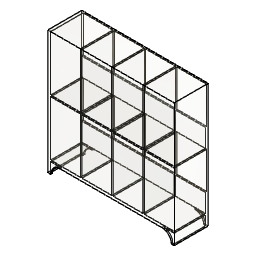
sorted_smarties_collector (Autodesk Fusion 360 design; units mm, degrees)
Autodesk Fusion 360 part; units mm, degrees
note: some values were not read from the file. Set by a fixed rule: which sketch regions a step uses.
sketch "Sorted Smarties Collector" plane through (0, 0, 0) normal (0, 1, 0) x (1, 0, 0)
  line L0 (0, 0) -> (268, 0)
  line L1 (268, 0) -> (268, -262)
  line L2 (268, -262) -> (0, -262)
  line L3 (0, -262) -> (0, 0)
  dimension "d1" = 268
  dimension "d41" = 262
  constraint horizontal L0
  constraint vertical L1
  constraint horizontal L2
  constraint vertical L3
  constraint coincident L0.start L3.end
  measures "d1" distance of L0.start L0.end
  measures "d41" distance of L0.end L1.end
extrude "Extrude1" add sketch "Sorted Smarties Collector" along normal blind 3
sketch "Smartie Collectors" plane through (0, 3, 0) normal (0, 1, 0) x (-1, 0, 0)
  line L0 (0, 262) -> (-268, 262)
  line L1 (-268, 262) -> (-268, 0)
  line L2 (-268, 0) -> (0, 0)
  line L3 (0, 0) -> (0, 262)
  line L4 (-265, 259) -> (-201.75, 259)
  line L5 (-201.75, 259) -> (-201.75, 142.5)
  line L6 (-201.75, 142.5) -> (-265, 142.5)
  line L7 (-265, 142.5) -> (-265, 259)
  line L8 (-198.75, 259) -> (-135.5, 259)
  line L9 (-135.5, 259) -> (-135.5, 142.5)
  line L10 (-135.5, 142.5) -> (-198.75, 142.5)
  line L11 (-198.75, 142.5) -> (-198.75, 259)
  line L12 (-132.5, 259) -> (-69.25, 259)
  line L13 (-69.25, 259) -> (-69.25, 142.5)
  line L14 (-69.25, 142.5) -> (-132.5, 142.5)
  line L15 (-132.5, 142.5) -> (-132.5, 259)
  line L16 (-66.25, 259) -> (-3, 259)
  line L17 (-3, 259) -> (-3, 142.5)
  line L18 (-3, 142.5) -> (-66.25, 142.5)
  line L19 (-66.25, 142.5) -> (-66.25, 259)
  line L20 (-265, 139.5) -> (-201.75, 139.5)
  line L21 (-201.75, 139.5) -> (-201.75, 23)
  line L22 (-201.75, 23) -> (-265, 23)
  line L23 (-265, 23) -> (-265, 139.5)
  line L24 (-198.75, 139.5) -> (-135.5, 139.5)
  line L25 (-135.5, 139.5) -> (-135.5, 23)
  line L26 (-135.5, 23) -> (-198.75, 23)
  line L27 (-198.75, 23) -> (-198.75, 139.5)
  line L28 (-132.5, 139.5) -> (-69.25, 139.5)
  line L29 (-69.25, 139.5) -> (-69.25, 23)
  line L30 (-69.25, 23) -> (-132.5, 23)
  line L31 (-132.5, 23) -> (-132.5, 139.5)
  line L32 (-66.25, 139.5) -> (-3, 139.5)
  line L33 (-3, 139.5) -> (-3, 23)
  line L34 (-3, 23) -> (-66.25, 23)
  line L35 (-66.25, 23) -> (-66.25, 139.5)
  line L36 (-265, 0) -> (-3, 0)
  line L37 (-3, 0) -> (-3, 20)
  line L38 (-3, 20) -> (-265, 20)
  line L39 (-265, 20) -> (-265, 0)
  dimension "d51" = 3
  dimension "d52" = 3
  dimension "d53" = 3
  dimension "d54" = 20
  dimension "d55" = 3
  dimension "d56" = 3
  dimension "d57" = 3
  dimension "d58" = 3
  dimension "d59" = 3
  dimension "d60" = 116.5
  dimension "d61" = 116.5
  dimension "d62" = 63.25
  dimension "d63" = 63.25
  dimension "d64" = 63.25
  dimension "d65" = 63.25
  constraint horizontal L4
  constraint vertical L5
  constraint horizontal L6
  constraint vertical L7
  constraint horizontal L8
  constraint vertical L9
  constraint horizontal L10
  constraint vertical L11
  constraint horizontal L12
  constraint vertical L13
  constraint horizontal L14
  constraint vertical L15
  constraint horizontal L16
  constraint vertical L17
  constraint horizontal L18
  constraint vertical L19
  constraint horizontal L20
  constraint vertical L21
  constraint horizontal L22
  constraint vertical L23
  constraint horizontal L24
  constraint vertical L25
  constraint horizontal L26
  constraint vertical L27
  constraint horizontal L28
  constraint vertical L29
  constraint horizontal L30
  constraint vertical L31
  constraint horizontal L32
  constraint vertical L33
  constraint horizontal L34
  constraint vertical L35
  constraint collinear L4 L8
  constraint collinear L8 L12
  constraint collinear L12 L16
  constraint collinear L6 L10
  constraint collinear L10 L14
  constraint collinear L14 L18
  constraint collinear L22 L26
  constraint collinear L26 L30
  constraint collinear L30 L34
  constraint collinear L20 L24
  constraint collinear L24 L28
  constraint collinear L28 L32
  constraint horizontal L36
  constraint vertical L37
  constraint horizontal L38
  constraint vertical L39
  constraint coincident L2 L36.start
  constraint collinear L23 L39
  constraint collinear L7 L23
  constraint collinear L5 L21
  constraint collinear L11 L27
  constraint collinear L9 L25
  constraint collinear L15 L31
  constraint collinear L13 L29
  constraint collinear L19 L35
  constraint collinear L17 L33
  constraint collinear L33 L37
  measures "d51" distance of L0 L4
  measures "d52" distance of L6 L20
  measures "d53" distance of L22 L38
  measures "d54" distance of L36 L38
  measures "d55" distance of L5 L11
  measures "d56" distance of L9 L15
  measures "d57" distance of L13 L19
  measures "d58" distance of L1 L7
  measures "d59" distance of L3 L17
  measures "d60" distance of L16.end L17.end
  measures "d61" distance of L32.end L33.end
  measures "d62" distance of L4.start L4.end
  measures "d63" distance of L8.start L8.end
  measures "d64" distance of L12.start L12.end
  measures "d65" distance of L16.start L16.end
extrude "Extrude2" add sketch "Smartie Collectors" along normal blind 69 contours L0 L1 L2 L3 L37 L38 L39
sketch "Front Panel" plane through (268, 0, 0) normal (1, 0, 0) x (0, 1, 0)
  line L0 (0, 262) -> (0, 0)
  line L1 (0, 0) -> (72, 0)
  line L2 (72, 0) -> (72, 262)
  line L3 (72, 262) -> (0, 262)
  line L4 (72, 262) -> (69, 262)
  line L5 (69, 262) -> (69, 0)
  line L6 (69, 0) -> (72, 0)
  line L7 (72, 0) -> (72, 262)
  dimension "d66" = 3
  constraint horizontal L4
  constraint vertical L5
  constraint horizontal L6
  constraint vertical L7
  constraint coincident L1 L5.end
  constraint coincident L2.end L3.start
  measures "d66" distance of L5.end L1.end
extrude "Extrude3" add sketch "Front Panel" against normal blind 268 contours L1 L2 L3 L4 L5 L6 L7
sketch "Front Openings" plane through (0, 72, 0) normal (0, 1, 0) x (-1, 0, 0)
  line L0 (-268, 0) -> (0, 0)
  line L1 (0, 0) -> (0, 262)
  line L2 (0, 262) -> (-268, 262)
  line L3 (-268, 262) -> (-268, 0)
  line L4 (0, 262) -> (-268, 262)
  line L5 (-198.75, 259) -> (-135.5, 259)
  line L6 (-265, 259) -> (-201.75, 259)
  line L7 (-201.75, 142.5) -> (-265, 142.5)
  line L8 (-265, 139.5) -> (-201.75, 139.5)
  line L9 (-201.75, 23) -> (-265, 23)
  line L10 (-135.5, 23) -> (-198.75, 23)
  line L11 (-69.25, 23) -> (-132.5, 23)
  line L12 (-3, 23) -> (-66.25, 23)
  line L13 (-132.5, 139.5) -> (-69.25, 139.5)
  line L14 (-198.75, 139.5) -> (-135.5, 139.5)
  line L15 (-135.5, 142.5) -> (-198.75, 142.5)
  line L16 (-69.25, 142.5) -> (-132.5, 142.5)
  line L17 (-3, 142.5) -> (-66.25, 142.5)
  line L18 (-66.25, 139.5) -> (-3, 139.5)
  line L19 (-132.5, 259) -> (-69.25, 259)
  line L20 (-66.25, 259) -> (-3, 259)
  line L21 (-3, 20) -> (-265, 20)
  line L22 (-3, 0) -> (-3, 20)
  line L23 (-265, 20) -> (-265, 0)
  line L24 (-265, 23) -> (-265, 139.5)
  line L25 (-201.75, 139.5) -> (-201.75, 23)
  line L26 (-198.75, 23) -> (-198.75, 139.5)
  line L27 (-135.5, 139.5) -> (-135.5, 23)
  line L28 (-132.5, 23) -> (-132.5, 139.5)
  line L29 (-69.25, 139.5) -> (-69.25, 23)
  line L30 (-66.25, 23) -> (-66.25, 139.5)
  line L31 (-3, 139.5) -> (-3, 23)
  line L32 (-265, 142.5) -> (-265, 259)
  line L33 (-201.75, 259) -> (-201.75, 142.5)
  line L34 (-198.75, 142.5) -> (-198.75, 259)
  line L35 (-135.5, 259) -> (-135.5, 142.5)
  line L36 (-132.5, 142.5) -> (-132.5, 259)
  line L37 (-69.25, 259) -> (-69.25, 142.5)
  line L38 (-66.25, 142.5) -> (-66.25, 259)
  line L39 (-3, 259) -> (-3, 142.5)
  line L40 (-265, 259) -> (-201.75, 259)
  line L41 (-201.75, 259) -> (-201.75, 181.3333)
  line L42 (-201.75, 181.3333) -> (-265, 181.3333)
  line L43 (-265, 181.3333) -> (-265, 259)
  line L44 (-198.75, 259) -> (-135.5, 259)
  line L45 (-135.5, 259) -> (-135.5, 181.3333)
  line L46 (-135.5, 181.3333) -> (-198.75, 181.3333)
  line L47 (-198.75, 181.3333) -> (-198.75, 259)
  line L48 (-132.5, 259) -> (-69.25, 259)
  line L49 (-69.25, 259) -> (-69.25, 181.3333)
  line L50 (-69.25, 181.3333) -> (-132.5, 181.3333)
  line L51 (-132.5, 181.3333) -> (-132.5, 259)
  line L52 (-66.25, 259) -> (-3, 259)
  line L53 (-3, 259) -> (-3, 181.3333)
  line L54 (-3, 181.3333) -> (-66.25, 181.3333)
  line L55 (-66.25, 181.3333) -> (-66.25, 259)
  line L56 (-265, 139.5) -> (-201.75, 139.5)
  line L57 (-201.75, 139.5) -> (-201.75, 61.8333)
  line L58 (-201.75, 61.8333) -> (-265, 61.8333)
  line L59 (-265, 61.8333) -> (-265, 139.5)
  line L60 (-198.75, 139.5) -> (-135.5, 139.5)
  line L61 (-135.5, 139.5) -> (-135.5, 61.8333)
  line L62 (-135.5, 61.8333) -> (-198.75, 61.8333)
  line L63 (-198.75, 61.8333) -> (-198.75, 139.5)
  line L64 (-132.5, 139.5) -> (-69.25, 139.5)
  line L65 (-69.25, 139.5) -> (-69.25, 61.8333)
  line L66 (-69.25, 61.8333) -> (-132.5, 61.8333)
  line L67 (-132.5, 61.8333) -> (-132.5, 139.5)
  line L68 (-66.25, 139.5) -> (-3, 139.5)
  line L69 (-3, 139.5) -> (-3, 61.8333)
  line L70 (-3, 61.8333) -> (-66.25, 61.8333)
  line L71 (-66.25, 61.8333) -> (-66.25, 139.5)
  line L72 (-3, 20) -> (-3, 0)
  line L73 (-3, 0) -> (-265, 0)
  line L74 (-265, 0) -> (-265, 20)
  dimension "d72" = 77.6667
  dimension "d73" = 77.6667
  constraint horizontal L40
  constraint vertical L41
  constraint horizontal L42
  constraint vertical L43
  constraint coincident L6.start L32.end
  constraint horizontal L44
  constraint vertical L45
  constraint horizontal L46
  constraint vertical L47
  constraint coincident L5.start L34.end
  constraint horizontal L48
  constraint vertical L49
  constraint horizontal L50
  constraint vertical L51
  constraint coincident L19.start L36.end
  constraint horizontal L52
  constraint vertical L53
  constraint horizontal L54
  constraint vertical L55
  constraint coincident L20.start L38.end
  constraint horizontal L56
  constraint vertical L57
  constraint horizontal L58
  constraint vertical L59
  constraint coincident L8.start L24.end
  constraint horizontal L60
  constraint vertical L61
  constraint horizontal L62
  constraint vertical L63
  constraint coincident L14.start L26.end
  constraint horizontal L64
  constraint vertical L65
  constraint horizontal L66
  constraint vertical L67
  constraint coincident L13.start L28.end
  constraint horizontal L68
  constraint vertical L69
  constraint horizontal L70
  constraint vertical L71
  constraint coincident L18.start L30.end
  constraint collinear L42 L46
  constraint collinear L46 L50
  constraint collinear L50 L54
  constraint collinear L58 L62
  constraint collinear L62 L66
  constraint collinear L66 L70
  constraint vertical L72
  constraint horizontal L73
  constraint vertical L74
  constraint coincident L22.start L72.end
  constraint coincident L21.end L23.start
  constraint collinear L33 L41
  constraint collinear L25 L57
  constraint collinear L35 L45
  constraint collinear L27 L61
  constraint collinear L37 L49
  constraint collinear L29 L65
  constraint collinear L39 L53
  constraint collinear L31 L69
  measures "d72" distance of L6.start L42.end
  measures "d73" distance of L8.start L58.end
extrude "Extrude4" cut sketch "Front Openings" against normal blind 3 contours L5 L34 L35 L44 L45 L46 L47 | L6 L32 L33 L40 L41 L42 L43 | L8 L24 L25 L56 L57 L58 L59 | L14 L26 L27 L60 L61 L62 L63 | L13 L28 L29 L64 L65 L66 L67 | L18 L30 L31 L68 L69 L70 L71 | L19 L36 L37 L48 L49 L50 L51 | L20 L38 L39 L52 L53 L54 L55
sketch "Slide Handle" plane through (0, 0, 0) normal (0, -1, 0) x (1, 0, 0)
  line L0 (0, 262) -> (0, 0)
  line L1 (0, 0) -> (268, 0)
  line L2 (268, 0) -> (268, 262)
  line L3 (3, 20) -> (265, 20)
  line L4 (3, 0) -> (3, 20)
  line L5 (265, 20) -> (265, 0)
  line L6 (265, 0) -> (3, 0)
  line L7 (268, 262) -> (268, 0)
  line L8 (0, 0) -> (0, 262)
  line L9 (0, 262) -> (268, 262)
  line L10 (268, 0) -> (0, 0)
  line L11 (26, 0) -> (242, 0)
  line L12 (242, 0) -> (242, 20)
  line L13 (242, 20) -> (26, 20)
  line L14 (26, 20) -> (26, 0)
  circle A0 centre (26, 0) radius 20
  circle A1 centre (242, 0) radius 20
  point P0 (268, 0)
  dimension "d77" = 20
  dimension "d78" = 40
  dimension "d79" = 40
  dimension "d80" = 26
  dimension "d81" = 26
  constraint horizontal L11
  constraint vertical L12
  constraint horizontal L13
  constraint vertical L14
  constraint coincident L1 L11.start
  constraint coincident L11.start L14.end
  constraint coincident L11.end L12.start
  measures "d77" distance of L11 L13
  measures "d78" diameter of A0
  measures "d79" diameter of A1
  measures "d80" distance of P0 L11.end
  measures "d81" distance of L0.end L11.start
extrude "Extrude5" cut sketch "Slide Handle" against normal blind 72 contours L1 L6 L10 L14 A0 | L1 L6 L10 L11 L14 A0 | L1 L3 L6 L10 L11 L13 A0 A1 | L1 L6 L10 L12 A1 | L1 L6 L10 L11 L12 A1
equation "d1 = width"
equation "polycarbonateThickness = 3 mm" comment "Thickness of the polycarbonate panels"
equation "d3 = polycarbonateThickness"
equation "collectorWidth = ( width - 5 * polycarbonateThickness ) / 4" comment "Width of a Smartie collector"
equation "d37 = collectorLength - polycarbonateThickness"
equation "collectorHeight = ( height - 3 * polycarbonateThickness - bottomHeight ) / 2" comment "Height of a Smartie Collector"
equation "height = 264 mm - tolerance" comment "Height of the Sorted Smarties Collector"
equation "d41 = height"
equation "bottomHeight = 20 mm" comment "Heigh of the botom part of the Sorted Smarties Collector"
equation "d51 = polycarbonateThickness"
equation "d52 = polycarbonateThickness"
equation "d53 = polycarbonateThickness"
equation "d54 = bottomHeight"
equation "d55 = polycarbonateThickness"
equation "d56 = polycarbonateThickness"
equation "d57 = polycarbonateThickness"
equation "d58 = polycarbonateThickness"
equation "d59 = polycarbonateThickness"
equation "d60 = collectorHeight"
equation "d62 = collectorWidth"
equation "d63 = collectorWidth"
equation "d64 = collectorWidth"
equation "d66 = polycarbonateThickness"
equation "d67 = -width"
equation "d69 = -polycarbonateThickness"
equation "openingHeight = collectorHeight * 2 / 3" comment "Height of the open part at the front of the Smartie collectors"
equation "d72 = openingHeight"
equation "d73 = openingHeight"
equation "d74 = -collectorLength"
equation "collectorLength = 72 mm" comment "Depth of the Sorted Smarties Collector Component"
equation "d80 = 2 * polycarbonateThickness + 20 mm"
equation "d81 = 2 * polycarbonateThickness + 20 mm"
equation "tolerance = 2 mm" comment "Tolerance to allow for easy motion"
equation "width = 270 mm - tolerance" comment "Width of the Sorted Smarties Component"
named bodies: "Sorted Smarties Collector"
